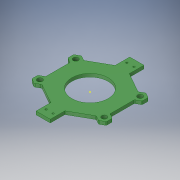
# Autodesk Inventor part: plate_fix
Saved by Autodesk Inventor 2019 (Build 230136000, 136)
## iProperties
Created: 2021-01-22
Part Number: plate_fix
Material: PET Plastic
Document SubType Name: Modeling
Designer: Juan M. Casillas
Density: 1.541 g/cm^3
Appearance: Smooth - Dark Forest Green
Author: Juan M. Casillas
## iProperties of the stored document plate_3DPrint.ipt
Created: 2021-01-22
Part Number: plate_3DPrint
Material: Genérico
Document SubType Name: Modeling
Designer: Juan M. Casillas
Density: 1 g/cm^3
Appearance: Valor por defecto
Author: Juan M. Casillas
Autodesk Inventor part; units mm, degrees
ref_plane "YZ Plane" through (0, 0, 0) normal (1, 0, 0) x (0, 1, 0)
ref_plane "XZ Plane" through (0, 0, 0) normal (0, 1, 0) x (-1, 0, 0)
ref_plane "XY Plane" through (0, 0, 0) normal (0, 0, 1) x (1, 0, 0)
sketch "Sketch1" plane through (0, 0, 0) normal (0, 1, 0) x (-1, 0, 0)
  line L0 (50, 27.85) -> (-50, 27.85) construction
  line L1 (-50, 27.85) -> (-50, -27.85) construction
  line L2 (-50, -27.85) -> (50, -27.85) construction
  line L3 (50, -27.85) -> (50, 27.85) construction
  line L4 (50, 27.85) -> (-50, -27.85) construction
  line L5 (-50, 27.85) -> (50, -27.85) construction
  circle A0 centre (50, 27.85) radius 4
  circle A1 centre (50, -27.85) radius 4
  circle A2 centre (-50, -27.85) radius 4
  circle A3 centre (-50, 27.85) radius 4
  line L6 (0, 0) -> (0, -29.6157) construction
  line L7 (0, 0) -> (0, 27.85) construction
  line L8 (0, 0) -> (50, 0) construction
  line L9 (0, 0) -> (-50, 0) construction
  circle A4 centre (0, 0) radius 30
  line L10 (-11, 35) -> (11, 35) construction
  line L11 (11, 35) -> (11, 50) construction
  line L12 (11, 50) -> (-11, 50)
  line L13 (-11, 50) -> (-11, 35) construction
  line L14 (-11, 35) -> (11, 50) construction
  line L15 (11, 35) -> (-11, 50) construction
  line L16 (-11, -50) -> (11, -50)
  line L17 (11, -50) -> (11, -35) construction
  line L18 (11, -35) -> (-11, -35) construction
  line L19 (-11, -35) -> (-11, -50) construction
  line L20 (-11, -50) -> (11, -35) construction
  line L21 (11, -50) -> (-11, -35) construction
  line L22 (-57.7942, -23.35) -> (-50, -18.85)
  line L23 (-50, -18.85) -> (-42.2058, -23.35) construction
  line L24 (-42.2058, -23.35) -> (-42.2058, -32.35) construction
  line L25 (-42.2058, -32.35) -> (-50, -36.85)
  line L26 (-50, -36.85) -> (-57.7942, -32.35)
  line L27 (-57.7942, -32.35) -> (-57.7942, -23.35)
  line L28 (-57.7942, 23.35) -> (-57.7942, 32.35)
  line L29 (-57.7942, 32.35) -> (-50, 36.85)
  line L30 (-50, 36.85) -> (-42.2058, 32.35)
  line L31 (-42.2058, 32.35) -> (-42.2058, 23.35) construction
  line L32 (-42.2058, 23.35) -> (-50, 18.85) construction
  line L33 (-50, 18.85) -> (-57.7942, 23.35)
  line L34 (42.2058, -23.35) -> (50, -18.85) construction
  line L35 (50, -18.85) -> (57.7942, -23.35)
  line L36 (57.7942, -23.35) -> (57.7942, -32.35)
  line L37 (57.7942, -32.35) -> (50, -36.85)
  line L38 (50, -36.85) -> (42.2058, -32.35)
  line L39 (42.2058, -32.35) -> (42.2058, -23.35) construction
  line L40 (50, 36.85) -> (57.7942, 32.35)
  line L41 (57.7942, 32.35) -> (57.7942, 23.35)
  line L42 (57.7942, 23.35) -> (50, 18.85)
  line L43 (50, 18.85) -> (42.2058, 23.35) construction
  line L44 (42.2058, 23.35) -> (42.2058, 32.35) construction
  line L45 (42.2058, 32.35) -> (50, 36.85)
  line L46 (-42.2058, -32.35) -> (-11, -50)
  line L47 (11, -50) -> (42.2058, -32.35)
  line L48 (-50, -18.85) -> (-50, 18.85)
  line L49 (-42.2058, 32.35) -> (-11, 50)
  line L50 (42.2058, 32.35) -> (11, 50)
  line L51 (50, 18.85) -> (50, -18.85)
  point P0 (0, 42.5)
  point P1 (0, -42.5)
  dimension "d0" = 100
  dimension "d1" = 55.7
  dimension "d2" = 8
  dimension "d3" = 8
  dimension "d4" = 8
  dimension "d5" = 8
  dimension "d6" = 60
  dimension "d11" = 22
  dimension "d12" = 15
  dimension "d13" = 35
  dimension "d14" = 22
  dimension "d15" = 15
  dimension "d16" = 35
  dimension "d20" = 18
  dimension "d21" = 18
  dimension "d22" = 18
  dimension "d25" = 18
  constraints: 104 end point, 11 parallel, 10 midpoint, 9 coincident, 5 centre point, 4 perpendicular, 3 horizontal, 2 collinear, 2 point on line, 52 other
  measures "d0" distance of L2.end L1.end
  measures "d1" distance of L1.end L0.end
  measures "d2" diameter of A0
  measures "d3" diameter of A1
  measures "d4" diameter of A2
  measures "d5" diameter of A3
  measures "d6" diameter of A4
  measures "d11" distance of L11.end L12.end
  measures "d12" distance of L10.end L11.end
  measures "d13" distance from line of L10 L6.start
  measures "d14" distance of L18.end L17.end
  measures "d15" distance of L17.end L16.end
  measures "d16" distance from line of L18 L6.start
  measures "d20" distance of L22.end L25.end
  measures "d21" distance of L29.end L32.end
  measures "d22" distance of L34.end L37.end
  measures "d25" distance of L40.start L42.end
extrude "Extrusion1" add sketch "Sketch1" along normal blind 3
sketch "Sketch2" plane through (0, 3, 0) normal (0, 1, 0) x (1, 0, 0)
  circle A0 centre (0, 0) radius 30 construction
  circle A1 centre (50, -27.85) radius 4 construction
  circle A2 centre (50, 27.85) radius 4 construction
  circle A3 centre (-50, 27.85) radius 4 construction
  circle A4 centre (-50, -27.85) radius 4 construction
  line L0 (11, 50) -> (-11, 50) construction
  line L1 (-11, 50) -> (-42.2058, 32.35) construction
  line L2 (-42.2058, 32.35) -> (-50, 36.85) construction
  line L3 (-50, 36.85) -> (-57.7942, 32.35) construction
  line L4 (-57.7942, 32.35) -> (-57.7942, 23.35) construction
  line L5 (-57.7942, 23.35) -> (-50, 18.85) construction
  line L6 (-50, 18.85) -> (-50, -18.85) construction
  line L7 (-50, -18.85) -> (-57.7942, -23.35) construction
  line L8 (-57.7942, -23.35) -> (-57.7942, -32.35) construction
  line L9 (-57.7942, -32.35) -> (-50, -36.85) construction
  line L10 (-50, -36.85) -> (-42.2058, -32.35) construction
  line L11 (-42.2058, -32.35) -> (-11, -50) construction
  line L12 (-11, -50) -> (11, -50) construction
  line L13 (11, -50) -> (42.2058, -32.35) construction
  line L14 (42.2058, -32.35) -> (50, -36.85) construction
  line L15 (50, -36.85) -> (57.7942, -32.35) construction
  line L16 (57.7942, -32.35) -> (57.7942, -23.35) construction
  line L17 (57.7942, -23.35) -> (50, -18.85) construction
  line L18 (50, -18.85) -> (50, 18.85) construction
  line L19 (50, 18.85) -> (57.7942, 23.35) construction
  line L20 (57.7942, 23.35) -> (57.7942, 32.35) construction
  line L21 (57.7942, 32.35) -> (50, 36.85) construction
  line L22 (50, 36.85) -> (42.2058, 32.35) construction
  line L23 (42.2058, 32.35) -> (11, 50) construction
  line L24 (-11, 37.577) -> (11, 37.577)
  line L25 (11, 37.577) -> (11, 50)
  line L26 (11, 50) -> (-11, 50)
  line L27 (-11, 50) -> (-11, 37.577)
  line L28 (-11, 37.577) -> (11, 50) construction
  line L29 (11, 37.577) -> (-11, 50) construction
  line L30 (11, 50) -> (-11, 50) projected
  line L31 (-11, -50) -> (11, -50)
  line L32 (11, -50) -> (11, -37.577)
  line L33 (11, -37.577) -> (-11, -37.577)
  line L34 (-11, -37.577) -> (-11, -50)
  point P0 (0, 43.7885)
  dimension "d28" = 22
  dimension "d29" = 12.423
  dimension "d30" = 12.423
  constraints: 20 end point, 4 parallel, 2 horizontal, 2 midpoint, 2 perpendicular, 1 collinear
  measures "d28" distance of L26.end L25.end
  measures "d29" distance of L25.end L24.end
  measures "d30" distance of L32.end L31.end
extrude "Extrusion2" add sketch "Sketch2" along normal blind 2
sketch "Sketch3" plane through (0, 0, 0) normal (0, -1, 0) x (1, 0, 0)
  line L0 (-11, -37.577) -> (11, -37.577) construction
  line L1 (11, -37.577) -> (11, -50) construction
  line L2 (11, -50) -> (-11, -50) construction
  line L3 (-11, -50) -> (-11, -37.577) construction
  line L4 (-11, 50) -> (11, 50) construction
  line L5 (11, 50) -> (11, 37.577) construction
  line L6 (11, 37.577) -> (-11, 37.577) construction
  line L7 (-11, 37.577) -> (-11, 50) construction
  line L8 (11, 50) -> (11, 37.577) construction
  line L9 (11, 43.7885) -> (-11, 43.7885) construction
  line L10 (-11, 37.577) -> (-11, 50) construction
  line L11 (0, 37.577) -> (0, 50) construction
  line L12 (-11, 50) -> (11, 50) construction
  line L13 (11, -37.577) -> (11, -50) construction
  line L14 (11, -43.7885) -> (-11, -43.7885) construction
  line L15 (-11, -50) -> (-11, -37.577) construction
  line L16 (11, -37.577) -> (-11, -37.577) construction
  line L17 (0, -37.577) -> (0, -50) construction
  line L18 (0, 43.7885) -> (5.5, 43.7885) construction
  line L19 (0, 43.7885) -> (-5.5, 43.7885) construction
  line L20 (0, -43.7885) -> (5.5, -43.7885) construction
  line L21 (0, -43.7885) -> (-5.5, -43.7885) construction
  point P0 (0, 0)
  dimension "d33" = 5.5
  dimension "d34" = 5.5
  dimension "d35" = 5.5
  dimension "d36" = 5.5
  constraints: 16 end point, 10 midpoint, 4 coincident, 4 point on line
  measures "d33" distance of L18.start L18.end
  measures "d34" distance of L18.start L19.end
  measures "d35" distance of L20.start L20.end
  measures "d36" distance of L20.start L21.end
hole "Hole1" [suppressed]
sketch "Sketch4" plane through (0, 0, 0) normal (0, -1, 0) x (1, 0, 0)
  circle A0 centre (5.5, 43.7885) radius 1.475 construction
  circle A1 centre (-5.5, 43.7885) radius 1.475 construction
  circle A2 centre (-5.5, -43.7885) radius 1.475 construction
  circle A3 centre (5.5, -43.7885) radius 1.475 construction
  point P0 (0, 0)
  constraints: 4 coincident
hole "Hole2" [suppressed]
fillet "Fillet1" radius 2 24 edges at (57.7942, 1.5, -23.35) (50, 1.5, -18.85) (57.7942, 1.5, -32.35) (50, 1.5, -36.85) (42.2058, 1.5, -32.35) (11, 1.5, -50) (-11, 1.5, -50) (-42.2058, 1.5, -32.35) (-50, 1.5, -36.85) (-57.7942, 1.5, -32.35) (-57.7942, 1.5, -23.35) (-50, 1.5, -18.85) (-50, 1.5, 18.85) (-57.7942, 1.5, 23.35) (-57.7942, 1.5, 32.35) (-50, 1.5, 36.85) (-42.2058, 1.5, 32.35) (-11, 1.5, 50) (11, 1.5, 50) (42.2058, 1.5, 32.35) (50, 1.5, 36.85) (57.7942, 1.5, 32.35) (57.7942, 1.5, 23.35) (50, 1.5, 18.85)
fillet "Fillet3" [suppressed]
sketch "Sketch6" plane through (0, 3, 0) normal (0, 1, 0) x (1, 0, 0)
  circle A0 centre (-50, -27.85) radius 4 construction
  circle A1 centre (-50, 27.85) radius 4 construction
  circle A2 centre (50, 27.85) radius 4 construction
  circle A3 centre (50, -27.85) radius 4 construction
  arc A4 (57.7942, -24.5047) -> (56.7942, -22.7726) centre (55.7942, -24.5047) ccw construction
  line L0 (56.7942, -22.7726) -> (51, -19.4274) construction
  arc A5 (50, -17.6953) -> (51, -19.4274) centre (52, -17.6953) ccw construction
  line L1 (50, -17.6953) -> (50, 17.6953) construction
  arc A6 (51, 19.4274) -> (50, 17.6953) centre (52, 17.6953) ccw construction
  line L2 (51, 19.4274) -> (56.7942, 22.7726) construction
  arc A7 (56.7942, 22.7726) -> (57.7942, 24.5047) centre (55.7942, 24.5047) ccw construction
  line L3 (57.7942, 24.5047) -> (57.7942, 31.1953) construction
  arc A8 (57.7942, 31.1953) -> (56.7942, 32.9274) centre (55.7942, 31.1953) ccw construction
  line L4 (56.7942, 32.9274) -> (51, 36.2726) construction
  arc A9 (51, 36.2726) -> (49, 36.2726) centre (50, 34.5406) ccw construction
  line L5 (49, 36.2726) -> (43.1956, 32.9215) construction
  arc A10 (41.211, 32.9127) -> (43.1956, 32.9215) centre (42.1956, 34.6535) ccw construction
  line L6 (41.211, 32.9127) -> (11.4582, 49.7408) construction
  arc A11 (11.4582, 49.7408) -> (11, 49.9295) centre (10.4736, 48) ccw construction
  line L7 (11, 49.9295) -> (11, 37.577) construction
  line L8 (11, 37.577) -> (-11, 37.577) construction
  line L9 (-11, 37.577) -> (-11, 49.9295) construction
  arc A12 (-11, 49.9295) -> (-11.4582, 49.7408) centre (-10.4736, 48) ccw construction
  line L10 (-11.4582, 49.7408) -> (-41.211, 32.9127) construction
  arc A13 (-43.1956, 32.9215) -> (-41.211, 32.9127) centre (-42.1956, 34.6535) ccw construction
  line L11 (-43.1956, 32.9215) -> (-49, 36.2726) construction
  arc A14 (-49, 36.2726) -> (-51, 36.2726) centre (-50, 34.5406) ccw construction
  line L12 (-51, 36.2726) -> (-56.7942, 32.9274) construction
  arc A15 (-56.7942, 32.9274) -> (-57.7942, 31.1953) centre (-55.7942, 31.1953) ccw construction
  line L13 (-57.7942, 31.1953) -> (-57.7942, 24.5047) construction
  arc A16 (-57.7942, 24.5047) -> (-56.7942, 22.7726) centre (-55.7942, 24.5047) ccw construction
  line L14 (-56.7942, 22.7726) -> (-51, 19.4274) construction
  arc A17 (-50, 17.6953) -> (-51, 19.4274) centre (-52, 17.6953) ccw construction
  line L15 (-50, 17.6953) -> (-50, -17.6953) construction
  arc A18 (-51, -19.4274) -> (-50, -17.6953) centre (-52, -17.6953) ccw construction
  line L16 (-51, -19.4274) -> (-56.7942, -22.7726) construction
  arc A19 (-56.7942, -22.7726) -> (-57.7942, -24.5047) centre (-55.7942, -24.5047) ccw construction
  line L17 (-57.7942, -24.5047) -> (-57.7942, -31.1953) construction
  arc A20 (-57.7942, -31.1953) -> (-56.7942, -32.9274) centre (-55.7942, -31.1953) ccw construction
  line L18 (-56.7942, -32.9274) -> (-51, -36.2726) construction
  arc A21 (-51, -36.2726) -> (-49, -36.2726) centre (-50, -34.5406) ccw construction
  line L19 (-49, -36.2726) -> (-43.1956, -32.9215) construction
  arc A22 (-41.211, -32.9127) -> (-43.1956, -32.9215) centre (-42.1956, -34.6535) ccw construction
  line L20 (-41.211, -32.9127) -> (-11.4582, -49.7408) construction
  arc A23 (-11.4582, -49.7408) -> (-11, -49.9295) centre (-10.4736, -48) ccw construction
  line L21 (-11, -49.9295) -> (-11, -37.577) construction
  line L22 (-11, -37.577) -> (11, -37.577) construction
  line L23 (11, -37.577) -> (11, -49.9295) construction
  arc A24 (11, -49.9295) -> (11.4582, -49.7408) centre (10.4736, -48) ccw construction
  line L24 (11.4582, -49.7408) -> (41.211, -32.9127) construction
  arc A25 (43.1956, -32.9215) -> (41.211, -32.9127) centre (42.1956, -34.6535) ccw construction
  line L25 (43.1956, -32.9215) -> (49, -36.2726) construction
  arc A26 (49, -36.2726) -> (51, -36.2726) centre (50, -34.5406) ccw construction
  line L26 (51, -36.2726) -> (56.7942, -32.9274) construction
  arc A27 (56.7942, -32.9274) -> (57.7942, -31.1953) centre (55.7942, -31.1953) ccw construction
  line L27 (57.7942, -31.1953) -> (57.7942, -24.5047) construction
  line L28 (-40, -27.85) -> (-40, 27.85) construction
  line L29 (-40, -27.85) -> (40, -27.85) construction
  line L30 (40, -27.85) -> (40, 27.85) construction
  line L31 (38.5, -27.85) -> (41.5, -27.85)
  line L32 (41.5, -27.85) -> (41.5, 27.85)
  line L33 (41.5, 27.85) -> (38.5, 27.85)
  line L34 (38.5, 27.85) -> (38.5, -27.85)
  line L35 (38.5, -27.85) -> (41.5, 27.85) construction
  line L36 (41.5, -27.85) -> (38.5, 27.85) construction
  line L37 (-41.5, -27.85) -> (-38.5, -27.85)
  line L38 (-38.5, -27.85) -> (-38.5, 27.85)
  line L39 (-38.5, 27.85) -> (-41.5, 27.85)
  line L40 (-41.5, 27.85) -> (-41.5, -27.85)
  line L41 (-41.5, -27.85) -> (-38.5, 27.85) construction
  line L42 (-38.5, -27.85) -> (-41.5, 27.85) construction
  line L43 (-10.4736, -50) -> (10.4736, -50) projected
  line L44 (10.4736, 50) -> (-10.4736, 50) projected
  line L45 (-11, -49.9295) -> (11, -49.9295)
  line L46 (11, -49.9295) -> (11, -69.6934)
  line L47 (11, -69.6934) -> (-11, -69.6934)
  line L48 (-11, -69.6934) -> (-11, -49.9295)
  line L49 (-11, 49.9295) -> (11, 49.9295)
  line L50 (11, 49.9295) -> (11, 69.6934)
  line L51 (11, 69.6934) -> (-11, 69.6934)
  line L52 (-11, 69.6934) -> (-11, 49.9295)
  circle A28 centre (-5.5, -43.7885) radius 1.475 construction
  circle A29 centre (5.5, -43.7885) radius 1.475 construction
  circle A30 centre (5.5, 43.7885) radius 1.475 construction
  circle A31 centre (-5.5, 43.7885) radius 1.475 construction
  circle A32 centre (5.5, -43.7885) radius 1.475 construction
  line L53 (-5.5, -43.7885) -> (5.5, -43.7885) construction
  line L54 (-11, 59.8115) -> (11, 59.8115) construction
  line L55 (-11, -59.8115) -> (11, -59.8115) construction
  circle A33 centre (-5.5, -43.7885) radius 2.825 construction
  line L56 (-5.5, -43.7885) -> (-5.5, -59.8115) construction
  line L57 (5.5, -43.7885) -> (5.5, -59.8115) construction
  circle A34 centre (-5.5, 43.7885) radius 2.825 construction
  line L58 (-5.5, 43.7885) -> (-5.5, 59.8115) construction
  line L59 (5.5, 43.7885) -> (5.5, 59.8115) construction
  line L60 (-11, -64.6934) -> (11, -64.6934) construction
  line L61 (-11, 64.6934) -> (11, 64.6934) construction
  point P0 (0, 0)
  point P1 (40, 0)
  point P2 (-40, 0)
  point P3 (5.5, 55.9169)
  point P4 (-5.5, -64.6934)
  point P5 (5.5, -64.6934)
  point P6 (-5.5, 64.6934)
  point P7 (5.5, 64.6934)
  dimension "d59" = 10
  dimension "d60" = 10
  dimension "d61" = 55.7
  dimension "d62" = 55.7
  dimension "d63" = 3
  dimension "d64" = 3
  dimension "d65" = 12.3525
  dimension "d66" = 19.764
  dimension "d67" = 19.764
  dimension "d102" = 5
  dimension "d103" = 5
  constraints: 64 end point, 17 point on line, 10 midpoint, 9 perpendicular, 8 parallel, 7 horizontal, 3 coincident, 2 vertical
  measures "d59" distance between parallel lines of L15 L28
  measures "d60" distance between parallel lines of L1 L30
  measures "d61" distance of L28.start L28.end
  measures "d62" distance of L29.end L30.end
  measures "d63" distance of L33.end L32.end
  measures "d64" distance of L39.end L38.end
  measures "d65" distance of L22.end L23.end
  measures "d66" distance of L45.end L46.end
  measures "d67" distance of L49.end L50.end
  measures "d102" distance between parallel lines of L47 L60
  measures "d103" distance between parallel lines of L51 L61
extrude "Extrusion4" add sketch "Sketch6" against normal up to surface (3 mm away) contours L45 L46 L47 L48 | L52 L51 L50 L49
extrude "Extrusion5" [suppressed]
extrude "Extrusion6" add sketch "Sketch6" along normal up to surface (2 mm away) contours L45 L46 L47 L48 | L52 L51 L50 L49
sketch "Sketch7" plane through (0, 5, 0) normal (0, 1, 0) x (1, 0, 0)
  arc A0 (11.4582, 49.7408) -> (11, 49.9295) centre (10.4736, 48) ccw construction
  line L0 (11, 49.9295) -> (11, 37.577) construction
  line L1 (11, 37.577) -> (-11, 37.577) construction
  line L2 (-11, 37.577) -> (-11, 49.9295) construction
  arc A1 (-11, 49.9295) -> (-11.4582, 49.7408) centre (-10.4736, 48) ccw construction
  arc A2 (-11.4582, -49.7408) -> (-11, -49.9295) centre (-10.4736, -48) ccw construction
  line L3 (-11, -49.9295) -> (-11, -37.577) construction
  line L4 (-11, -37.577) -> (11, -37.577) construction
  line L5 (11, -37.577) -> (11, -49.9295) construction
  arc A3 (11, -49.9295) -> (11.4582, -49.7408) centre (10.4736, -48) ccw construction
  line L6 (-10.4736, -50) -> (10.4736, -50)
  line L7 (10.4736, 50) -> (-10.4736, 50)
  line L8 (-11, -49.9295) -> (11, -49.9295)
  line L9 (11, -49.9295) -> (11, -62.282)
  line L10 (11, -62.282) -> (-11, -62.282)
  line L11 (-11, -62.282) -> (-11, -49.9295)
  line L12 (-11, 49.9295) -> (11, 49.9295)
  line L13 (11, 49.9295) -> (11, 62.282)
  line L14 (11, 62.282) -> (-11, 62.282)
  line L15 (-11, 62.282) -> (-11, 49.9295)
  circle A4 centre (-5.5, -43.7885) radius 1.475 construction
  circle A5 centre (5.5, -43.7885) radius 1.475 construction
  circle A6 centre (5.5, 43.7885) radius 1.475 construction
  circle A7 centre (-5.5, 43.7885) radius 1.475 construction
  circle A8 centre (5.5, -43.7885) radius 1.475 construction
  line L16 (-5.5, -43.7885) -> (5.5, -43.7885) construction
  line L17 (-11, 56.1057) -> (11, 56.1057) construction
  line L18 (-11, -56.1057) -> (11, -56.1057) construction
  circle A9 centre (-5.5, -43.7885) radius 2.825 construction
  line L19 (-5.5, -43.7885) -> (-5.5, -56.1057) construction
  line L20 (5.5, -43.7885) -> (5.5, -56.1057) construction
  circle A10 centre (-5.5, 43.7885) radius 2.825 construction
  line L21 (-5.5, 43.7885) -> (-5.5, 56.1057) construction
  line L22 (5.5, 43.7885) -> (5.5, 56.1057) construction
  point P0 (0, 0)
  point P1 (0, 0)
  point P2 (0, 0)
  point P3 (5.5, 55.9169)
  dimension "d74" = 12.3525
  dimension "d75" = 12.3525
  dimension "d76" = 12.3525
  constraints: 46 end point, 11 centre point, 8 point on circle, 6 perpendicular, 6 point on line, 4 midpoint, 4 parallel, 3 coincident, 3 horizontal
  measures "d74" distance of L5.start L5.end
  measures "d75" distance of L8.end L10.start
  measures "d76" distance of L13.start L13.end
hole "Hole3" [suppressed]
hole "Hole4" [suppressed]
sketch "Sketch8" plane through (0, 0, 0) normal (0, -1, 0) x (1, 0, 0)
  circle A0 centre (-5.5, 56.1057) radius 1.475 projected
  circle A1 centre (5.5, 56.1057) radius 1.475 projected
  circle A2 centre (5.5, -55.9169) radius 1.475 projected
  circle A3 centre (-5.5, -56.1057) radius 1.475 projected
  point P0 (0, 0)
  constraints: 4 coincident
fillet "Fillet5" [suppressed]
sketch "Sketch10" plane through (0, 5, 0) normal (0, 1, 0) x (1, 0, 0)
  circle A0 centre (-50, -27.85) radius 4 construction
  circle A1 centre (-50, 27.85) radius 4 construction
  circle A2 centre (50, 27.85) radius 4 construction
  circle A3 centre (50, -27.85) radius 4 construction
  arc A4 (57.7942, -24.5047) -> (56.7942, -22.7726) centre (55.7942, -24.5047) ccw construction
  line L0 (56.7942, -22.7726) -> (51, -19.4274) construction
  arc A5 (50, -17.6953) -> (51, -19.4274) centre (52, -17.6953) ccw construction
  line L1 (50, -17.6953) -> (50, 17.6953) construction
  arc A6 (51, 19.4274) -> (50, 17.6953) centre (52, 17.6953) ccw construction
  line L2 (51, 19.4274) -> (56.7942, 22.7726) construction
  arc A7 (56.7942, 22.7726) -> (57.7942, 24.5047) centre (55.7942, 24.5047) ccw construction
  line L3 (57.7942, 24.5047) -> (57.7942, 31.1953) construction
  arc A8 (57.7942, 31.1953) -> (56.7942, 32.9274) centre (55.7942, 31.1953) ccw construction
  line L4 (56.7942, 32.9274) -> (51, 36.2726) construction
  arc A9 (51, 36.2726) -> (49, 36.2726) centre (50, 34.5406) ccw construction
  line L5 (49, 36.2726) -> (43.1956, 32.9215) construction
  arc A10 (41.211, 32.9127) -> (43.1956, 32.9215) centre (42.1956, 34.6535) ccw construction
  line L6 (41.211, 32.9127) -> (11.4582, 49.7408) construction
  arc A11 (11.4582, 49.7408) -> (11, 49.9295) centre (10.4736, 48) ccw construction
  line L7 (11, 49.9295) -> (11, 37.577) construction
  line L8 (11, 37.577) -> (-11, 37.577) construction
  line L9 (-11, 37.577) -> (-11, 49.9295) construction
  arc A12 (-11, 49.9295) -> (-11.4582, 49.7408) centre (-10.4736, 48) ccw construction
  line L10 (-11.4582, 49.7408) -> (-41.211, 32.9127) construction
  arc A13 (-43.1956, 32.9215) -> (-41.211, 32.9127) centre (-42.1956, 34.6535) ccw construction
  line L11 (-43.1956, 32.9215) -> (-49, 36.2726) construction
  arc A14 (-49, 36.2726) -> (-51, 36.2726) centre (-50, 34.5406) ccw construction
  line L12 (-51, 36.2726) -> (-56.7942, 32.9274) construction
  arc A15 (-56.7942, 32.9274) -> (-57.7942, 31.1953) centre (-55.7942, 31.1953) ccw construction
  line L13 (-57.7942, 31.1953) -> (-57.7942, 24.5047) construction
  arc A16 (-57.7942, 24.5047) -> (-56.7942, 22.7726) centre (-55.7942, 24.5047) ccw construction
  line L14 (-56.7942, 22.7726) -> (-51, 19.4274) construction
  arc A17 (-50, 17.6953) -> (-51, 19.4274) centre (-52, 17.6953) ccw construction
  line L15 (-50, 17.6953) -> (-50, -17.6953) construction
  arc A18 (-51, -19.4274) -> (-50, -17.6953) centre (-52, -17.6953) ccw construction
  line L16 (-51, -19.4274) -> (-56.7942, -22.7726) construction
  arc A19 (-56.7942, -22.7726) -> (-57.7942, -24.5047) centre (-55.7942, -24.5047) ccw construction
  line L17 (-57.7942, -24.5047) -> (-57.7942, -31.1953) construction
  arc A20 (-57.7942, -31.1953) -> (-56.7942, -32.9274) centre (-55.7942, -31.1953) ccw construction
  line L18 (-56.7942, -32.9274) -> (-51, -36.2726) construction
  arc A21 (-51, -36.2726) -> (-49, -36.2726) centre (-50, -34.5406) ccw construction
  line L19 (-49, -36.2726) -> (-43.1956, -32.9215) construction
  arc A22 (-41.211, -32.9127) -> (-43.1956, -32.9215) centre (-42.1956, -34.6535) ccw construction
  line L20 (-41.211, -32.9127) -> (-11.4582, -49.7408) construction
  arc A23 (-11.4582, -49.7408) -> (-11, -49.9295) centre (-10.4736, -48) ccw construction
  line L21 (-11, -49.9295) -> (-11, -37.577) construction
  line L22 (-11, -37.577) -> (11, -37.577) construction
  line L23 (11, -37.577) -> (11, -49.9295) construction
  arc A24 (11, -49.9295) -> (11.4582, -49.7408) centre (10.4736, -48) ccw construction
  line L24 (11.4582, -49.7408) -> (41.211, -32.9127) construction
  arc A25 (43.1956, -32.9215) -> (41.211, -32.9127) centre (42.1956, -34.6535) ccw construction
  line L25 (43.1956, -32.9215) -> (49, -36.2726) construction
  arc A26 (49, -36.2726) -> (51, -36.2726) centre (50, -34.5406) ccw construction
  line L26 (51, -36.2726) -> (56.7942, -32.9274) construction
  arc A27 (56.7942, -32.9274) -> (57.7942, -31.1953) centre (55.7942, -31.1953) ccw construction
  line L27 (57.7942, -31.1953) -> (57.7942, -24.5047) construction
  circle A28 centre (0, 0) radius 32 construction
  line L28 (-40, -27.85) -> (-40, 27.85) construction
  line L29 (-40, -27.85) -> (40, -27.85) construction
  line L30 (40, -27.85) -> (40, 27.85) construction
  line L31 (38.5, -27.85) -> (41.5, -27.85)
  line L32 (41.5, -27.85) -> (41.5, 27.85)
  line L33 (41.5, 27.85) -> (38.5, 27.85)
  line L34 (38.5, 27.85) -> (38.5, -27.85)
  line L35 (38.5, -27.85) -> (41.5, 27.85) construction
  line L36 (41.5, -27.85) -> (38.5, 27.85) construction
  line L37 (-41.5, -27.85) -> (-38.5, -27.85)
  line L38 (-38.5, -27.85) -> (-38.5, 27.85)
  line L39 (-38.5, 27.85) -> (-41.5, 27.85)
  line L40 (-41.5, 27.85) -> (-41.5, -27.85)
  line L41 (-41.5, -27.85) -> (-38.5, 27.85) construction
  line L42 (-38.5, -27.85) -> (-41.5, 27.85) construction
  line L43 (-10.4736, -50) -> (10.4736, -50)
  line L44 (10.4736, 50) -> (-10.4736, 50)
  line L45 (-11, -49.9295) -> (11, -49.9295)
  line L46 (11, -49.9295) -> (11, -69.6934)
  line L47 (11, -69.6934) -> (-11, -69.6934)
  line L48 (-11, -69.6934) -> (-11, -49.9295)
  line L49 (-11, 49.9295) -> (11, 49.9295)
  line L50 (11, 49.9295) -> (11, 69.6934)
  line L51 (11, 69.6934) -> (-11, 69.6934)
  line L52 (-11, 69.6934) -> (-11, 49.9295)
  circle A29 centre (-5.5, -41.7885) radius 1.475 construction
  circle A30 centre (5.5, -43.7885) radius 1.475 construction
  circle A31 centre (5.5, 43.7885) radius 1.475 construction
  circle A32 centre (-5.5, 43.7885) radius 1.475 construction
  circle A33 centre (5.5, -41.7885) radius 1.475 construction
  line L53 (-5.5, -41.7885) -> (5.5, -41.7885) construction
  line L54 (-11, 59.8115) -> (11, 59.8115) construction
  line L55 (-11, -59.8115) -> (11, -59.8115) construction
  circle A34 centre (-5.5, -41.7885) radius 2.825 construction
  line L56 (-5.5, -41.7885) -> (-5.5, -59.8115) construction
  line L57 (5.5, -41.7885) -> (5.5, -59.8115) construction
  circle A35 centre (-5.5, 43.7885) radius 2.825 construction
  line L58 (-5.5, 43.7885) -> (-5.5, 59.8115) construction
  line L59 (5.5, 43.7885) -> (5.5, 59.8115) construction
  line L60 (-11, -62.6934) -> (11, -62.6934) construction
  line L61 (-11, 62.6934) -> (11, 62.6934) construction
  point P0 (40, 0)
  point P1 (-40, 0)
  point P2 (5.5, 55.9169)
  point P3 (-5.5, -62.6934)
  point P4 (5.5, -62.6934)
  point P5 (-5.5, 62.6934)
  point P6 (5.5, 62.6934)
  dimension "d104" = 10
  dimension "d105" = 10
  dimension "d106" = 55.7
  dimension "d107" = 55.7
  dimension "d108" = 3
  dimension "d109" = 3
  dimension "d110" = 12.3525
  dimension "d111" = 19.764
  dimension "d112" = 19.764
  dimension "d113" = 7
  dimension "d114" = 7
  constraints: 124 end point, 48 point on circle, 36 centre point, 17 point on line, 10 midpoint, 9 perpendicular, 8 parallel, 7 horizontal, 3 coincident, 2 vertical
  measures "d104" distance between parallel lines of L15 L28
  measures "d105" distance between parallel lines of L1 L30
  measures "d106" distance of L28.start L28.end
  measures "d107" distance of L29.end L30.end
  measures "d108" distance of L34.start L35.end
  measures "d109" distance of L39.end L39.start
  measures "d110" distance of L23.start L23.end
  measures "d111" distance of L46.start L46.end
  measures "d112" distance of L49.end L51.start
  measures "d113" distance between parallel lines of L47 L60
  measures "d114" distance between parallel lines of L51 L61
hole "Hole6" at (-5.5, 5, -62.6934) at (5.5, 5, -62.6934) at (-5.5, 5, 62.6934) at (5.5, 5, 62.6934) direction (0, -1, 0) diameter 2.95 end through all
sketch "Sketch11" plane through (0, 0, 0) normal (0, -1, 0) x (1, 0, 0)
  circle A0 centre (-5.5, 62.6934) radius 1.475 projected
  circle A1 centre (5.5, 62.6934) radius 1.475 projected
  circle A2 centre (-5.5, -62.6934) radius 1.475 projected
  circle A3 centre (5.5, -62.6934) radius 1.475 projected
  point P0 (0, 0)
  constraints: 4 coincident
hole "Hole7" at (-5.5, 0, 62.6934) at (5.5, 0, 62.6934) at (-5.5, 0, -62.6934) at (5.5, 0, -62.6934) direction (0, 1, 0) diameter 5.65 depth 2.95
sketch "Sketch12" plane through (0, 5, 0) normal (0, 1, 0) x (1, 0, 0)
  circle A0 centre (-5.5, 62.6934) radius 1.475 construction
  circle A1 centre (5.5, 62.6934) radius 1.475 construction
  line L0 (-11, 69.6934) -> (-11, 37.577) construction
  line L1 (-11, 37.577) -> (11, 37.577) construction
  line L2 (11, 37.577) -> (11, 69.6934) construction
  line L3 (-11, 69.6934) -> (11, 69.6934) construction
  point P0 (0, 0)
  dimension "d129" = 32.1164
  dimension "d130" = 22
  dimension "d131" = 7
  measures "d129" distance of L1.end L2.end
  measures "d130" distance of L0.start L2.end
  measures "d131" distance from line of A1.centre L3
sketch "Sketch13" plane through (0, 5, 0) normal (0, 1, 0) x (1, 0, 0)
  circle A0 centre (5.5, -62.6934) radius 1.475 construction
  circle A1 centre (-5.5, -62.6934) radius 1.475 construction
  line L0 (11, -69.6934) -> (-11, -69.6934) construction
  point P0 (0, 0)
  dimension "d132" = 7
  measures "d132" distance from line of L0 A0.centre
thicken "Thicken1" operation add thickness 3 both sides no extend neighbours yes toward (0, 0, 1) faces at (3.6667, 3.3333, 69.6934)
thicken "Thicken2" operation add thickness 3 both sides no extend neighbours yes toward (0, 0, -1) faces at (3.6667, 3.3333, -69.6934)
thicken "Thicken3" operation add thickness 2 both sides no extend neighbours yes toward (0, 1, 0) faces at (43.3333, 3, 0)
thicken "Thicken4" operation add thickness 2 both sides no extend neighbours yes toward (0.9967573, 0, -0.0804666) faces at (-29.9027, 1.6667, 2.414)
thicken "Thicken5" operation add thickness 0.2 both sides no extend neighbours yes toward (-0.9967573, 0, 0.0804666) faces at (-27.9092, 1.6667, 2.2531)
sketch "Sketch5" plane through (0, 3, 0) normal (0, 1, 0) x (1, 0, 0)
  circle A0 centre (0, 0) radius 45
  circle A1 centre (0, 0) radius 38
  circle A2 centre (0, 0) radius 30 projected
  line L0 (0, 0) -> (0, 21.8801) construction
  line L1 (0, 0) -> (-31.0093, 32.6102) construction
  line L2 (0, 0) -> (-15.5636, 42.2229) construction
  line L3 (0, 0) -> (-24.1039, 38) construction
  line L4 (-24.1039, 38) -> (-24.1039, -38) construction
  line L5 (-24.1039, -38) -> (24.1039, -38) construction
  line L6 (24.1039, -38) -> (24.1039, 38) construction
  line L7 (24.1039, 38) -> (-24.1039, 38) construction
  line L8 (-11, 37.577) -> (11, 37.577) construction
  line L9 (0, 0) -> (24.1039, 38) construction
  line L10 (0, 0) -> (24.1039, -38) construction
  line L11 (0, 0) -> (-24.1039, -38) construction
  line L12 (-24.1039, -38) -> (-20.3544, -32.0889)
  line L13 (-24.1039, 38) -> (-20.3544, 32.0889)
  line L14 (24.1039, -38) -> (20.3544, -32.0889)
  line L15 (24.1039, 38) -> (20.3544, 32.0889)
  dimension "d54" = 7
  dimension "d55" = 15
  constraints: 30 end point, 5 point on line, 4 point on circle, 2 collinear, 2 perpendicular, 1 centre point, 1 parallel, 1 vertical, 9 other
equation "\"d2\" = d4"
equation "\"d3\" = d4"
equation "\"d5\" = d4"
equation "\"d14\" = d11"
equation "\"d15\" = d12"
equation "\"d16\" = d13"
equation "\"d21\" = d20"
equation "\"d22\" = d20"
equation "\"d25\" = d20"
equation "\"d60\" = d59"
equation "\"d66\" = 1.6 * d65"
equation "\"d67\" = d66"
equation "\"d75\" = d74"
equation "\"d76\" = d75"
equation "\"d105\" = d104"
equation "\"d111\" = 1.6 * d110"
equation "\"d112\" = d111"
equation "\"d113\" = d114"
body "Solid1"
